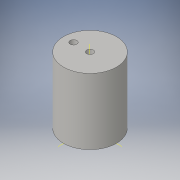
# Autodesk Inventor part: Pneumatickolben_Zylinder
Saved by Autodesk Inventor 2016 (Build 200138000, 138)
## iProperties
Created: 2019-05-08
Part Number: Pneumatickolben_Zylinder
Material: Generisch
Document SubType Name: Modeling
Designer: Teilnehmer
Density: 1 g/cm^3
Appearance: Vorgabe
Author: Teilnehmer
Autodesk Inventor part; units mm, degrees
ref_plane "YZ Plane" through (0, 0, 0) normal (1, 0, 0) x (0, 1, 0)
ref_plane "XZ Plane" through (0, 0, 0) normal (0, 1, 0) x (-1, 0, 0)
ref_plane "XY Plane" through (0, 0, 0) normal (0, 0, 1) x (1, 0, 0)
sketch "Skizze1" plane through (0, 0, 0) normal (0, 0, 1) x (1, 0, 0)
  circle A0 centre (0, 0) radius 4
  dimension "d0" = 8
  constraints: 1 centre point, 1 coincident
  measures "d0" diameter of A0
extrude "Extrusion1" add sketch "Skizze1" along normal blind 10
sketch "Skizze2" plane through (0, 0, 10) normal (0, 0, 1) x (1, 0, 0)
  circle A0 centre (0, 0) radius 3.5
  dimension "d3" = 7
  constraints: 1 centre point, 1 coincident
  measures "d3" diameter of A0
extrude "Extrusion2" cut sketch "Skizze2" against normal blind 9
sketch "Skizze3" plane through (0, 0, 10) normal (0, 0, 1) x (1, 0, 0)
  circle A0 centre (0, 0) radius 3.5
  constraints: 1 centre point, 1 coincident
extrude "Extrusion3" add sketch "Skizze3" against normal blind 1
sketch "Skizze4" plane through (0, 0, 10) normal (0, 0, 1) x (1, 0, 0)
  circle A0 centre (0, 0) radius 0.5
  dimension "d8" = 1
  constraints: 1 centre point, 1 coincident
  measures "d8" diameter of A0
extrude "Extrusion4" cut sketch "Skizze4" against normal blind 1
sketch "Skizze5" plane through (0, 0, 10) normal (0, 0, 1) x (1, 0, 0)
  circle A0 centre (-2.5, 0) radius 0.5
  circle A1 centre (0, 0) radius 4 projected
  line L0 (-5.6, 0) -> (5.6, 0) projected
  dimension "d11" = 1
  dimension "d12" = 2.5
  dimension "d13" = 0
  constraints: 1 centre point
  measures "d11" diameter of A0
  measures "d12" distance of point (0, 0) A0.centre
  measures "d13" distance from line of A0.centre L0
extrude "Extrusion5" cut sketch "Skizze5" against normal blind 1 contours L0 A0 | A0 L0
sketch "Skizze6" plane through (0, 0, 0) normal (0, 0, -1) x (-1, 0, 0)
  circle A0 centre (2.5, 0) radius 0.5
  line L0 (5.6, 0) -> (-5.6, 0) projected
  point P0 (0, 0)
  dimension "d16" = 1
  dimension "d17" = 2.5
  dimension "d18" = 0
  constraints: 1 centre point
  measures "d16" diameter of A0
  measures "d17" distance of point (0, 0) A0.centre
  measures "d18" distance from line of L0 A0.centre
extrude "Extrusion6" cut sketch "Skizze6" against normal blind 1
